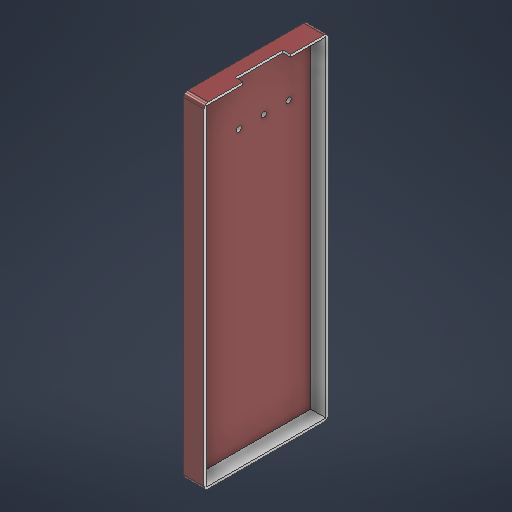
# Autodesk Inventor part: cDAQ_Lid_Box
Saved by Autodesk Inventor 2027 (Build 310192000, 192)
## iProperties
Created: 2026-05-08
Part Number: cDAQ_Lid_Box
Material: Generic
Document SubType Name: Modeling
Designer: giese
Density: 1 g/cm^3
Appearance: Default
Author: giese
Autodesk Inventor part; units mm, degrees
ref_plane "YZ Plane" through (0, 0, 0) normal (1, 0, 0) x (0, 1, 0)
ref_plane "XZ Plane" through (0, 0, 0) normal (0, 1, 0) x (-1, 0, 0)
ref_plane "XY Plane" through (0, 0, 0) normal (0, 0, 1) x (1, 0, 0)
sketch "Sketch1" plane through (0, 0, 0) normal (1, 0, 0) x (0, 1, 0)
  line L0 (50.7569, 48.4212) -> (-198.7981, 48.4212)
  line L1 (-198.7981, 48.4212) -> (-198.7981, -44.2888)
  line L2 (-198.7981, -44.2888) -> (50.7569, -44.2888)
  line L3 (50.7569, -44.2888) -> (50.7569, 48.4212)
  point P0 (0, 0)
  dimension "d0" = 92.71
  dimension "d1" = 249.555
  constraints: 8 end point, 2 parallel, 1 horizontal, 1 perpendicular
  measures "d0" distance of L2.end L0.start
  measures "d1" distance of L0.start L0.end
extrude "Extrusion1" add sketch "Sketch1" along normal blind 15.24
sketch "Sketch2" plane through (15.24, 0, 0) normal (1, 0, 0) x (0, 0, -1)
  line L0 (-46.5162, 48.8519) -> (42.3838, 48.8519)
  line L1 (42.3838, 48.8519) -> (42.3838, -196.8931)
  line L2 (42.3838, -196.8931) -> (-46.5162, -196.8931)
  line L3 (-46.5162, -196.8931) -> (-46.5162, 48.8519)
  line L4 (-48.4212, 50.7569) -> (-48.4212, -198.7981) projected
  line L5 (-48.4212, -198.7981) -> (44.2888, -198.7981) projected
  point P0 (0, 0)
  dimension "d4" = 88.9
  dimension "d5" = 245.745
  dimension "d6" = 1.905
  dimension "d7" = 1.905
  constraints: 8 end point, 2 parallel, 1 horizontal, 1 perpendicular
  measures "d4" distance of L0.start L0.end
  measures "d5" distance of L0.end L1.end
  measures "d6" distance between parallel lines of L4 L3
  measures "d7" distance between parallel lines of L5 L2
extrude "Extrusion2" cut sketch "Sketch2" against normal blind 11.43
sketch "Sketch3" plane through (0, 0, 0) normal (-1, 0, 0) x (0, 0, 1)
  circle A0 centre (-26.0008, 10.5233) radius 2
  line L0 (-44.2888, -198.7981) -> (-44.2888, 50.7569) projected
  line L1 (-44.2888, 50.7569) -> (48.4212, 50.7569) projected
  circle A1 centre (-7.502, 10.5233) radius 2
  circle A2 centre (10.9969, 10.5233) radius 2
  point P0 (0, 0)
  dimension "d10" = 18.288
  dimension "d11" = 40.2336
  dimension "d12" = 40.2336
  dimension "d13" = 18.4988
  dimension "d14" = 4
  dimension "d15" = 4
  dimension "d16" = 40.2336
  dimension "d17" = 18.4988
  dimension "d18" = 36.9976
  dimension "d21" = 4
  constraints: 3 centre point
  measures "d10" distance from line of L0 A0.centre
  measures "d11" distance from line of L1 A0.centre
  measures "d12" distance from line of L1 A1.centre
  measures "d13" distance of A0.centre A1.centre
  measures "d14" diameter of A1
  measures "d15" diameter of A2
  measures "d16" distance from line of L1 A2.centre
  measures "d17" distance of A1.centre A2.centre
  measures "d18" distance of A0.centre A2.centre
  measures "d21" diameter of A0
extrude "Extrusion3" cut sketch "Sketch3" against normal blind 3.81
sketch "Sketch6" plane through (0, 50.7569, 48.4212) normal (0, 1, 0) x (1, 0, 0)
  line L0 (15.24, 1.905) -> (15.24, 90.805) projected
  line L1 (9.4234, 28.9459) -> (15.24, 28.9459)
  line L2 (15.24, 28.9459) -> (15.24, 64.516)
  line L3 (15.24, 64.516) -> (9.4234, 64.516)
  line L4 (9.4234, 64.516) -> (9.4234, 28.9459)
  line L5 (0, 92.71) -> (15.24, 92.71) projected
  point P0 (0, 48.4212)
  point P1 (12.3317, 64.516)
  point P2 (12.3317, 28.9459)
  dimension "d30" = 5.8166
  dimension "d31" = 35.5701
  dimension "d32" = 28.194
  constraints: 8 end point, 2 midpoint, 2 parallel, 1 horizontal, 1 perpendicular, 1 point on line
  measures "d30" distance between parallel lines of L0 L4
  measures "d31" distance of point (12.332, 64.516) point (12.332, 28.946)
  measures "d32" distance between parallel lines of L5 L3
extrude "Extrusion5" cut sketch "Sketch6" against normal blind 3.81
fillet "Fillet1" radius 3.175 4 edges at (7.62, 50.7569, -44.2888) (7.62, 50.7569, 48.4212) (7.62, -198.7981, 48.4212) (7.62, -198.7981, -44.2888)
body "Solid1"
